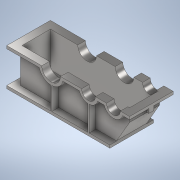
# Autodesk Inventor part: МПСТ Корпус
Saved by Autodesk Inventor 2022.1 (Build 261234020, 234B)
## iProperties
Created: 2021-12-02
Part Number: МПСТ Корпус
Material: Сталь, углеродистая
Document SubType Name: Modeling
Designer: Алексанян Г.
Density: 7.85 g/cm^3
Appearance: С умеренной полировкой
Author: Алексанян Г.
Autodesk Inventor part; units mm, degrees
ref_plane "YZ Plane" through (0, 0, 0) normal (1, 0, 0) x (0, 1, 0)
ref_plane "XZ Plane" through (0, 0, 0) normal (0, 1, 0) x (-1, 0, 0)
ref_plane "XY Plane" through (0, 0, 0) normal (0, 0, 1) x (1, 0, 0)
sketch "Эскиз1" plane through (0, 0, 0) normal (0, 1, 0) x (-1, 0, 0)
  line L0 (493, -175) -> (-493, -175)
  line L1 (-493, -175) -> (-493, 175)
  line L2 (-493, 175) -> (493, 175)
  line L3 (493, 175) -> (493, -175)
  line L4 (493, -175) -> (-493, 175) construction
  line L5 (-493, -175) -> (493, 175) construction
  point P0 (0, 0)
  dimension "d0" = 986
  dimension "d1" = 350
  constraints: 12 end point, 2 midpoint, 2 parallel, 1 horizontal, 1 perpendicular
  measures "d0" distance of L0.start L0.end
  measures "d1" distance of L2.end L0.start
extrude "Выдавливание1" add sketch "Эскиз1" against normal blind 300
sketch "Эскиз2" plane through (0, -300, 0) normal (0, -1, 0) x (1, 0, 0)
  line L0 (493, 175) -> (-493, 175) projected
  line L1 (-493, 175) -> (-493, -175) projected
  line L2 (-493, -175) -> (493, -175) projected
  line L3 (493, -175) -> (493, 175) projected
  line L4 (-438, 120) -> (438, 120)
  line L5 (438, 120) -> (438, -120)
  line L6 (438, -120) -> (-438, -120)
  line L7 (-438, -120) -> (-438, 120)
  point P0 (0, 0)
  dimension "d4" = 55
  constraints: 8 end point, 3 other
  measures "d4" distance between parallel lines of L0 L4
extrude "Выдавливание2" cut sketch "Эскиз2" against normal blind 277.5
sketch "Эскиз4" plane through (-493, 0, 175) normal (0, 0, 1) x (1, 0, 0)
  line L0 (0, 0) -> (986, 0) projected
  line L1 (986, 0) -> (827.2287, -275)
  line L2 (986, 0) -> (1303.5426, 0) construction
  line L3 (931, -300) -> (55, -300) projected
  line L4 (931, -95.2628) -> (931, -300)
  line L5 (931, -300) -> (931, -22.5) projected
  line L6 (827.2287, -275) -> (827.2287, -300)
  line L7 (827.2287, -300) -> (931, -300)
  point P0 (493, 0)
  dimension "d10" = 120
  dimension "d13" = 25
  constraints: 10 end point, 3 point on line, 2 horizontal, 1 equal length, 1 vertical
  measures "d10" angle of L1 L2
  measures "d13" distance from line of L3 L1.end
extrude "Выдавливание3" cut sketch "Эскиз4" against normal through all
sketch "Эскиз5" plane through (0, -300, 0) normal (0, -1, 0) x (1, 0, 0)
  line L0 (-493, -175) -> (-493, 175) construction
  line L1 (493, -175) -> (-493, -175) construction
  line L2 (493, 175) -> (493, -175) construction
  line L3 (-493, 175) -> (493, 175) construction
  line L4 (438, 120) -> (-438, 120) construction
  line L5 (438, -120) -> (438, 120) construction
  line L6 (-438, -120) -> (438, -120) construction
  line L7 (-438, 120) -> (-438, -120) construction
  line L8 (-493, 175) -> (493, 175) projected
  line L9 (334.2287, 175) -> (-493, 175)
  line L10 (-493, -175) -> (-493, 175) projected
  line L11 (-493, 175) -> (-493, -175)
  line L12 (-493, -175) -> (334.2287, -175)
  line L13 (493, -175) -> (-493, -175) projected
  line L14 (334.2287, 175) -> (334.2287, -175)
  point P0 (0, 0)
  point P1 (334.2287, 120)
  constraints: 8 end point, 3 point on line, 2 collinear, 1 perpendicular
extrude "Выдавливание5" add sketch "Эскиз5" against normal blind 22.5
shell "Оболочка1" thickness 6 removed faces 1 at (-164.3333, 0, -58.3333)
sketch "Эскиз6" plane through (-487, -16.5, 169) normal (0, 1, 0) x (1, 0, 0)
  line L0 (0, 338) -> (0, 0) projected
  line L1 (0, 0) -> (974, 0) projected
  line L2 (974, 0) -> (974, 338) projected
  line L3 (974, 338) -> (0, 338) projected
  line L4 (919, 55) -> (55, 55) projected
  line L5 (55, 55) -> (55, 283) projected
  line L6 (55, 283) -> (919, 283) projected
  line L7 (919, 283) -> (919, 55) projected
  point P0 (487, 169)
extrude "Выдавливание6" add sketch "Эскиз6" along normal up to surface (16.5 mm away)
sketch "Эскиз7" plane through (-487, -294, -169) normal (0, 1, 0) x (1, 0, 0)
  line L0 (815.2287, 0) -> (815.2287, -338) projected
  line L1 (0, 0) -> (815.2287, 0) projected
  line L2 (0, -338) -> (0, 0) projected
  line L3 (815.2287, -338) -> (0, -338) projected
  point P0 (487, -169)
extrude "Выдавливание7" add sketch "Эскиз7" along normal up to surface (10.5 mm away)
sketch "Эскиз8" plane through (-493, 0, 175) normal (0, 0, 1) x (1, 0, 0)
  line L0 (0, 0) -> (986, 0) projected
  line L1 (986, 0) -> (986, -22.5) projected
  circle A0 centre (856, 0) radius 55
  circle A1 centre (856, 0) radius 77.5
  circle A2 centre (356, 0) radius 75
  circle A3 centre (356, 0) radius 97.5
  circle A4 centre (656, 0) radius 55
  circle A5 centre (656, 0) radius 77.5
  point P0 (493, 0)
  point P1 (986, -11.25)
  point P2 (778.5, 0)
  point P3 (933.5, 0)
  point P4 (911, 0)
  point P5 (801, 0)
  point P6 (578.5, 0)
  point P7 (733.5, 0)
  point P8 (711, 0)
  point P9 (601, 0)
  point P10 (258.5, 0)
  point P11 (453.5, 0)
  point P12 (431, 0)
  point P13 (281, 0)
  dimension "d21" = 130
  dimension "d22" = 200
  dimension "d23" = 300
  dimension "d24" = 110
  dimension "d25" = 22.5
  dimension "d26" = 150
  dimension "d27" = 22.5
  dimension "d28" = 110
  dimension "d29" = 22.5
  constraints: 6 centre point, 3 coincident, 3 point on line, 1 midpoint
  measures "d21" horizontal distance of point (986, -11.25) point (856, 0)
  measures "d22" distance of point (656, 0) point (856, 0)
  measures "d23" distance of point (356, 0) point (656, 0)
  measures "d24" diameter of A0
  measures "d25" radial gap between concentric circles of A0 A1
  measures "d26" diameter of A2
  measures "d27" radial gap between concentric circles of A2 A3
  measures "d28" diameter of A4
  measures "d29" radial gap between concentric circles of A4 A5
extrude "Выдавливание8" add sketch "Эскиз8" against normal up to surface (55 mm away) contours L0 A3 A2 | L0 A5 A4 | L0 A1 A0 picked at (445.6692, -4.6252) picked at (691.0844, -60.3286) picked at (891.0844, -60.3286)
extrude "Выдавливание9" cut sketch "Эскиз8" against normal up to surface (61 mm away) contours A2 L0 | L0 A2 | A4 L0 | L0 A4 | A0 L0 | L0 A0
sketch "Эскиз9" plane through (493, 0, -175) normal (0, 0, -1) x (-1, 0, 0)
  line L0 (0, 0) -> (986, 0) projected
  circle A0 centre (130, 0) radius 55
  circle A1 centre (630, 0) radius 75
  circle A2 centre (330, 0) radius 75
  circle A3 centre (130, 0) radius 77.5
  circle A4 centre (330, 0) radius 97.5
  circle A5 centre (630, 0) radius 97.5
  point P0 (493, 0)
  point P1 (532.5, 0)
  point P2 (727.5, 0)
  point P3 (705, 0)
  point P4 (555, 0)
  point P5 (232.5, 0)
  point P6 (427.5, 0)
  point P7 (405, 0)
  point P8 (255, 0)
  point P9 (52.5, 0)
  point P10 (207.5, 0)
  point P11 (185, 0)
  point P12 (75, 0)
  dimension "d34" = 130
  dimension "d35" = 200
  dimension "d36" = 300
  dimension "d37" = 110
  dimension "d38" = 150
  dimension "d39" = 150
  dimension "d40" = 22.5
  dimension "d41" = 22.5
  dimension "d42" = 22.5
  constraints: 6 centre point, 3 coincident, 3 horizontal alignment
  measures "d34" distance of L0.start point (130, 0)
  measures "d35" distance of point (130, 0) point (330, 0)
  measures "d36" distance of point (330, 0) point (630, 0)
  measures "d37" diameter of A0
  measures "d38" diameter of A1
  measures "d39" diameter of A2
  measures "d40" radial gap between concentric circles of A0 A3
  measures "d41" radial gap between concentric circles of A2 A4
  measures "d42" radial gap between concentric circles of A1 A5
extrude "Выдавливание10" add sketch "Эскиз9" against normal up to surface (55 mm away) contours L0 A3 A0 | L0 A4 A2 | L0 A5 A1 picked at (94.9156, -60.3286) picked at (419.6692, -4.6252) picked at (719.6692, -4.6252)
extrude "Выдавливание11" cut sketch "Эскиз9" against normal up to surface (61 mm away) contours A0 L0 | L0 A0 | A2 L0 | L0 A2 | A1 L0 | L0 A1
sketch "Эскиз10" plane through (-493, 0, 175) normal (0, 0, 1) x (1, 0, 0)
  line L0 (356, -129.0257) -> (356, -213.661)
  line L1 (656, -124.2861) -> (656, -204.1819)
  point P0 (493, 0)
  constraints: 4 end point, 2 vertical
rib "Ребро жесткости1" sketch "Эскиз10" thickness 10 direction (0, 0, -1) end up to next extend profile yes curves L0 L1
sketch "Эскиз11" plane through (-212, 0, -175) normal (0, 0, -1) x (-1, 0, 0)
  line L0 (-375, -125.9374) -> (-375, -199.7394)
  line L1 (-75, -121.1978) -> (-75, -208.5414)
  arc A0 (-430, 0) -> (-320, 0) centre (-375, 0) ccw projected
  arc A1 (-150, 0) -> (0, 0) centre (-75, 0) ccw projected
  point P0 (-212, 0)
  point P1 (-375, -162.8384)
  point P2 (-375, -55)
  point P3 (-75, -75)
  constraints: 4 end point, 2 point on circle, 2 vertical, 2 vertical alignment, 1 midpoint
rib "Ребро жесткости2" sketch "Эскиз11" thickness 10 direction (0, 0, 1) end up to next extend profile yes curves L0 L1
sketch "Эскиз12" plane through (0, 0, 0) normal (0, 0, 1) x (1, 0, 0)
  line L0 (-231.8683, -22.5) -> (-493, -22.5) projected
  line L1 (-493, -22.5) -> (-493, -55.5)
  line L2 (-491, -57.5) -> (-474.799, -57.5)
  line L3 (-472.799, -55.5) -> (-472.799, -53.3284)
  line L4 (-438, -277.5) -> (-438, -22.5) projected
  line L5 (-438, -67.5) -> (-467.9497, -37.5503)
  line L6 (-438, -67.5) -> (-395.6447, -67.5) construction
  arc A0 (-467.9497, -37.5503) -> (-477.8492, -47.4497) centre (-472.8995, -42.5) ccw
  line L7 (-477.8492, -47.4497) -> (-473.3848, -51.9142)
  arc A1 (-493, -55.5) -> (-491, -57.5) centre (-491, -55.5) ccw
  arc A2 (-474.799, -57.5) -> (-472.799, -55.5) centre (-474.799, -55.5) ccw
  arc A3 (-472.799, -53.3284) -> (-473.3848, -51.9142) centre (-474.799, -53.3284) ccw
  point P0 (0, 0)
  point P1 (-493, -57.5)
  point P2 (-472.799, -57.5)
  point P3 (-472.799, -52.5)
  dimension "d59" = 35
  dimension "d60" = 135
  dimension "d61" = 45
  dimension "d63" = 7
  dimension "d64" = 15
  dimension "d65" = 5
  dimension "d66" = 2
  constraints: 12 end point, 8 point on circle, 8 tangent, 7 point on line, 4 centre point, 2 equal radius, 2 perpendicular, 1 equal length, 1 horizontal, 1 parallel, 1 vertical
  measures "d59" distance of L0.end point (-493, -57.5)
  measures "d60" angle of L6 L5
  measures "d61" distance from line of L5.start L0
  measures "d63" radius of A0
  measures "d64" vertical distance of point (-472.799, -57.5) A0.centre
  measures "d65" distance of point (-472.799, -57.5) point (-472.799, -52.5)
  measures "d66" radius of A1
extrude "Выдавливание12" add sketch "Эскиз12" along normal mid plane 40
mirror "Зеркальное отражение1" about plane through (0, 0, 0) normal (1, 0, 0) of "Выдавливание12"
ref_plane "РабПлоскость1" through (0, 0, 0) normal (1, 0, 0) x (0, 1, 0)
